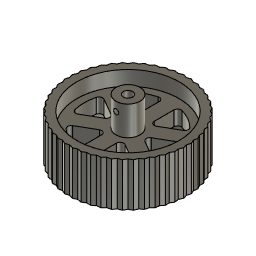
wheel (Autodesk Fusion 360 design; units mm, degrees)
Autodesk Fusion 360 part; units mm, degrees
sketch "Sketch1" plane through (0, 0, 0) normal (0, 0, 1) x (1, 0, 0)
  circle A0 centre (0, 0) radius 3.25
  circle A1 centre (0, 0) radius 40
  circle A2 centre (0, 0) radius 8.25
  circle A3 centre (0, 0) radius 35
  line L0 (0, 0) -> (0, 35) construction
  line L1 (0, 0) -> (30.3109, 17.5) construction
  arc A4 (20.905, 21.517) -> (8.1818, 28.8627) centre (0, 0) ccw
  line L2 (5, 12.9904) -> (5, 26.4575)
  line L3 (5, 34.641) -> (5, 35)
  line L4 (8.75, 10.8253) -> (20.4129, 17.5589)
  line L5 (27.5, 21.6506) -> (27.8109, 21.8301)
  arc A5 (8.1818, 28.8627) -> (5, 26.4575) centre (7.5, 26.4575) ccw
  arc A6 (20.4129, 17.5589) -> (20.905, 21.517) centre (19.1629, 19.7239) ccw
  arc A7 (5, 12.9904) -> (8.75, 10.8253) centre (7.5, 12.9904) ccw
  line L6 (-5, 12.9904) -> (-5, 26.4575)
  arc A8 (-8.1818, 28.8627) -> (-20.905, 21.517) centre (0, 0) ccw
  line L7 (-8.75, 10.8253) -> (-20.4129, 17.5589)
  arc A9 (-8.75, 10.8253) -> (-5, 12.9904) centre (-7.5, 12.9904) ccw
  arc A10 (-20.905, 21.517) -> (-20.4129, 17.5589) centre (-19.1629, 19.7239) ccw
  arc A11 (-5, 26.4575) -> (-8.1818, 28.8627) centre (-7.5, 26.4575) ccw
  line L8 (-13.75, 2.1651) -> (-25.4129, 8.8986)
  arc A12 (-29.0868, 7.3457) -> (-29.0868, -7.3457) centre (0, 0) ccw
  line L9 (-13.75, -2.1651) -> (-25.4129, -8.8986)
  arc A13 (-13.75, -2.1651) -> (-13.75, 2.1651) centre (-15, 0) ccw
  arc A14 (-29.0868, -7.3457) -> (-25.4129, -8.8986) centre (-26.6629, -6.7336) ccw
  arc A15 (-25.4129, 8.8986) -> (-29.0868, 7.3457) centre (-26.6629, 6.7336) ccw
  line L10 (-8.75, -10.8253) -> (-20.4129, -17.5589)
  arc A16 (-20.905, -21.517) -> (-8.1818, -28.8627) centre (0, 0) ccw
  line L11 (-5, -12.9904) -> (-5, -26.4575)
  arc A17 (-5, -12.9904) -> (-8.75, -10.8253) centre (-7.5, -12.9904) ccw
  arc A18 (-8.1818, -28.8627) -> (-5, -26.4575) centre (-7.5, -26.4575) ccw
  arc A19 (-20.4129, -17.5589) -> (-20.905, -21.517) centre (-19.1629, -19.7239) ccw
  line L12 (5, -12.9904) -> (5, -26.4575)
  arc A20 (8.1818, -28.8627) -> (20.905, -21.517) centre (0, 0) ccw
  line L13 (8.75, -10.8253) -> (20.4129, -17.5589)
  arc A21 (8.75, -10.8253) -> (5, -12.9904) centre (7.5, -12.9904) ccw
  arc A22 (20.905, -21.517) -> (20.4129, -17.5589) centre (19.1629, -19.7239) ccw
  arc A23 (5, -26.4575) -> (8.1818, -28.8627) centre (7.5, -26.4575) ccw
  line L14 (13.75, -2.1651) -> (25.4129, -8.8986)
  arc A24 (29.0868, -7.3457) -> (29.0868, 7.3457) centre (0, 0) ccw
  line L15 (13.75, 2.1651) -> (25.4129, 8.8986)
  arc A25 (13.75, 2.1651) -> (13.75, -2.1651) centre (15, 0) ccw
  arc A26 (29.0868, 7.3457) -> (25.4129, 8.8986) centre (26.6629, 6.7336) ccw
  arc A27 (25.4129, -8.8986) -> (29.0868, -7.3457) centre (26.6629, -6.7336) ccw
  dimension "d1" = 6.5
  dimension "d2" = 80
  dimension "d3" = 16.5
  dimension "d4" = 70
  dimension "d9" = 60
  dimension "d12" = 2.5
  dimension "d14" = 360
  constraint coincident A0.centre A1.centre
  constraint concentric A1 A3
  constraint vertical L0
  constraint coincident A3 L0.end
  constraint coincident A3 L1.end
  constraint parallel L0 L2
  constraint parallel L1 L4
  constraint coincident A3 L3.start
  constraint collinear L2 L3
  constraint coincident A3 L5.start
  constraint collinear L4 L5
  constraint tangent A4 A5
  constraint tangent L2 A5
  constraint tangent A4 A6
  constraint tangent L4 A6
  constraint equal A5 A6
  constraint tangent L2 A7
  constraint tangent L4 A7
  constraint equal A5 A7
  measures "d1" diameter of A0
  measures "d2" diameter of A1
  measures "d3" diameter of A2
  measures "d4" diameter of A3
  measures "d9" angle of L0 L1
  measures "d12" radius of A5
extrude "Extrude1" add sketch "Sketch1" along normal mid plane 30 contours A1
extrude "Extrude5" add sketch "Sketch1" along normal mid plane 10 contours A3
extrude "Extrude6" add sketch "Sketch1" along normal blind 25 and the other way blind 5 contours A2
sketch "Sketch3" plane through (0, 0, 0) normal (0, 1, 0) x (1, 0, 0)
  line L0 (-8.25, -25) -> (8.25, -25)
  line L1 (-40, -15) -> (40, -15)
  line L2 (0, -25) -> (0, -15) construction
  line L3 (0, -15) -> (0, -17)
  circle A0 centre (0, -18.75) radius 1.75
  dimension "d30" = 2
  dimension "d31" = 3.5
  constraint midpoint L0 L2.start
  constraint midpoint L1 L2.end
  constraint perpendicular L1 L3
  constraint coincident L3.end A0
  measures "d30" distance of L2.end L3.end
  measures "d31" diameter of A0
extrude "Extrude7" cut sketch "Sketch3" along normal mid plane 16.5
sketch "Sketch4" plane through (0, 0, -15) normal (0, 0, -1) x (1, 0, 0)
  circle A0 centre (0, 0) radius 35
  circle A1 centre (0, 0) radius 40
  line L0 (0, 0) -> (5.221, 39.6578)
  line L1 (0, 0) -> (40, 0) construction
  line L2 (0, 0) -> (0, 40)
  line L3 (0, 40) -> (5.221, 39.6578)
  line L4 (2.6105, 39.8289) -> (2.6759, 40.8268) construction
  line L5 (2.6759, 40.8268) -> (0, 40)
  line L6 (2.6759, 40.8268) -> (5.221, 39.6578)
  circle A2 centre (0, 0) radius 40
  dimension "d34" = 82.5
  dimension "d35" = 1
  constraint horizontal L1
  constraint coincident A0.centre A1.centre
  constraint coincident A1 L0.end
  constraint coincident A1 L2.end
  constraint vertical L2
  constraint midpoint L3 L4.start
  constraint perpendicular L3 L4
  measures "d34" angle of L0 L1
  measures "d35" distance of L4.start L4.end
extrude "Extrude8" add sketch "Sketch4" against normal blind 30 contours A1 L5 L6 A2
pattern_circular "C-Pattern1" count 48 over 360 about axis through (0, 0, 1.75) along (0, 0, 1) of "Extrude8"
move_body "Move1" bodies 1 to x (1, 0, 0) y (0, 1, 0) z (0, 0, 1) at (0, 0, 15)
equation "d3 = 10 mm + 6.5 mm"
equation "d27 = 15 mm + ( 20 / 2 ) * 1 mm"
equation "d32 = 10 mm + 6.5 mm"
equation "d34 = 90 deg - ( ( 360 / 48 ) * 1 deg )"
